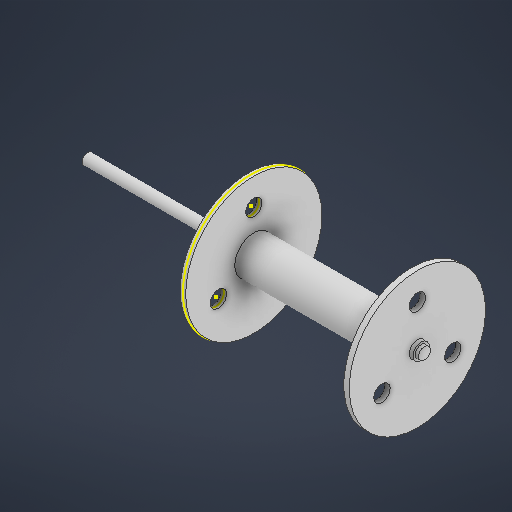
# Autodesk Inventor part: roller
Saved by Autodesk Inventor 2026.1 (Build 301233020, 233B)
## iProperties
Created: 2025-12-30
Part Number: roller
Material: Generic
Document SubType Name: Modeling
Designer: Austin Ngobeni
Density: 1 g/cm^3
Appearance: Default
Author: Austin Ngobeni
Autodesk Inventor part; units mm, degrees
ref_plane "YZ Plane" through (0, 0, 0) normal (1, 0, 0) x (0, 1, 0)
ref_plane "XZ Plane" through (0, 0, 0) normal (0, 1, 0) x (-1, 0, 0)
ref_plane "XY Plane" through (0, 0, 0) normal (0, 0, 1) x (1, 0, 0)
sketch "Sketch1" plane through (0, 0, 0) normal (1, 0, 0) x (0, 1, 0)
  circle A0 centre (0, 0) radius 35
  circle A1 centre (0, 0) radius 125
  circle A2 centre (0, 0) radius 10 construction
  line L0 (-8.55, -5.1863) -> (-8.7665, 4.8113)
  line L1 (-8.7665, 4.8113) -> (-0.2165, 9.9977)
  line L2 (-0.2165, 9.9977) -> (8.55, 5.1863)
  line L3 (8.55, 5.1863) -> (8.7665, -4.8113)
  line L4 (8.7665, -4.8113) -> (0.2165, -9.9977)
  line L5 (0.2165, -9.9977) -> (-8.55, -5.1863)
  circle A3 centre (0, 0) radius 15
  circle A4 centre (0, 0) radius 75 construction
  circle A5 centre (75, 0) radius 15
  circle A6 centre (-37.5, 64.9519) radius 15
  circle A7 centre (-37.5, -64.9519) radius 15
  circle A8 centre (0, 0) radius 11
  dimension "d2" = 20
  dimension "d12" = 150
  dimension "d0" = 70
  dimension "d1" = 250
  dimension "d3" = 30
  dimension "d13" = 30
  dimension "d16" = 360
  dimension "d20" = 22
  constraints: 12 end point, 7 centre point, 7 coincident, 1 horizontal alignment, 25 other
  measures "d0" diameter of A0
  measures "d1" diameter of A1
  measures "d3" diameter of A3
  measures "d13" diameter of A5
  measures "d20" diameter of A8
extrude "Extrusion1" add sketch "Sketch1" along normal mid plane 10 contours A0 | A1 | L0 L1 L2 L3 L4 L5 | A3 | A5 | A6 | A7 | A8
extrude "Extrusion2" add sketch "Sketch1" against normal blind 300 contours A0
extrude "Extrusion3" add sketch "Sketch1" along normal blind 15 contours L0 L1 L2 L3 L4 L5
extrude "Extrusion4" add sketch "Sketch1" along normal blind 12 contours A3 | A8
extrude "Extrusion5" cut sketch "Sketch1" along normal through all both and the other way through all contours A5 | A6 | A7
extrude "Extrusion6" add sketch "Sketch1" along normal blind 18 contours L0 L1 L2 L3 L4 L5 | A8
sketch "Sketch2" plane through (-300, 0, 0) normal (-1, 0, 0) x (0, 0, 1)
  circle A0 centre (0, 0) radius 125 projected
  circle A1 centre (0, 75) radius 15 projected
  circle A2 centre (-64.9519, -37.5) radius 15 projected
  circle A3 centre (64.9519, -37.5) radius 15 projected
  circle A4 centre (0, 0) radius 15 projected
  circle A5 centre (0, 0) radius 10 projected
  line L0 (4.8113, -8.7665) -> (-5.1863, -8.55) projected
  line L1 (-5.1863, -8.55) -> (-9.9977, 0.2165) projected
  line L2 (-9.9977, 0.2165) -> (-4.8113, 8.7665) projected
  line L3 (-4.8113, 8.7665) -> (5.1863, 8.55) projected
  line L4 (5.1863, 8.55) -> (9.9977, -0.2165) projected
  line L5 (9.9977, -0.2165) -> (4.8113, -8.7665) projected
extrude "Extrusion7" add sketch "Sketch2" along normal mid plane 10 contours A0
extrude "Extrusion8" add sketch "Sketch2" along normal blind 300 contours A5 L4 | L3 A5 | L4 L5 L0 L1 L2 L3 | A5 L5 | L2 A5 | A5 L0 | L1 A5
extrude "Extrusion10" add sketch "Sketch2" along normal blind 12 contours A4 | A5 L4 | L3 A5 | L4 L5 L0 L1 L2 L3 | A5 L5 | L2 A5 | A5 L0 | L1 A5
body "Solid1"
